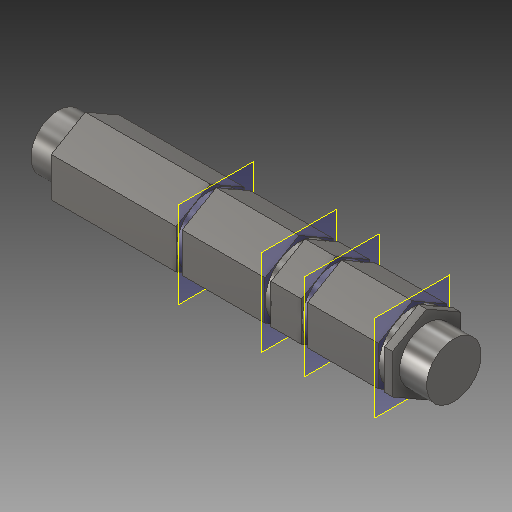
# Autodesk Inventor part: Shaft Jr
Saved by Autodesk Inventor 2019.4 (Build 234330000, 330)
## iProperties
Created: 2019-12-11
Part Number: Shaft Jr
Material: Steel, Mild
Document SubType Name: Modeling
Designer: admin
Density: 7.85 g/cm^3
Appearance: Semi-Polished
Mass: 72.1586 g
Surface Area: 33.9276 cm^2
Volume: 9.19217 cm^3
Author: admin
Autodesk Inventor part; units mm, degrees
ref_plane "YZ Plane" through (0, 0, 0) normal (1, 0, 0) x (0, 1, 0)
ref_plane "XZ Plane" through (0, 0, 0) normal (0, 1, 0) x (-1, 0, 0)
ref_plane "XY Plane" through (0, 0, 0) normal (0, 0, 1) x (1, 0, 0)
sketch "Sketch1" plane through (0, 0, 0) normal (0, 0, 1) x (1, 0, 0)
  line L0 (0, 0) -> (0, 5)
  line L1 (0, 5) -> (5, 5)
  line L2 (5, 5) -> (5, 15)
  line L3 (5, 15) -> (67.6, 15)
  line L4 (67.6, 15) -> (67.6, 5)
  line L5 (67.6, 5) -> (72.6, 5)
  line L6 (72.6, 5) -> (72.6, 0)
  line L7 (72.6, 0) -> (0, 0)
  dimension "d0" = 5
  dimension "d1" = 15
  dimension "d2" = 5
  dimension "d3" = 5
  dimension "d4" = 62.6
  constraints: 16 end point, 6 perpendicular, 2 point on line, 1 vertical
  measures "d0" distance of L5.end L6.end
  measures "d1" distance between parallel lines of L7 L3
  measures "d2" distance of L0.end L1.end
  measures "d3" distance of L4.end L5.end
  measures "d4" distance of L2.end L3.end
revolve "Revolution1" add sketch "Sketch1" angle 360 about axis through (72.6, 0, 0) along (-1, 0, 0)
sketch "Sketch2" plane through (67.6, 0, 0) normal (1, 0, 0) x (0, 0, -1)
  line L0 (0, 7.2169) -> (6.25, 3.6084)
  line L1 (6.25, 3.6084) -> (6.25, -3.6084)
  line L2 (6.25, -3.6084) -> (0, -7.2169)
  line L3 (0, -7.2169) -> (-6.25, -3.6084)
  line L4 (-6.25, -3.6084) -> (-6.25, 3.6084)
  line L5 (-6.25, 3.6084) -> (0, 7.2169)
  circle A0 centre (0, 0) radius 15 projected
  dimension "d6" = 12.5
  constraints: 12 end point, 1 coincident, 13 other
  measures "d6" distance between parallel lines of L1 L4
extrude "Extrusion1" cut sketch "Sketch2" against normal through all
ref_plane "Work Plane1" through (29, -3.6084, -6.25) normal (-1, 0, 0) x (0, 0, 1)
sketch "Sketch3" plane through (29, -3.6084, -6.25) normal (-1, 0, 0) x (0, 0, 1)
  circle A0 centre (6.25, 3.6084) radius 6.2
  line L0 (12.5, 7.2169) -> (6.25, 10.8253) projected
  circle A1 centre (6.25, 3.6084) radius 7.2169
  dimension "d10" = 12.4
  constraints: 2 coincident, 1 centre point, 1 vertical alignment, 2 other
  measures "d10" diameter of A0
extrude "Extrusion2" cut sketch "Sketch3" along normal blind 1.1
ref_plane "Work Plane2" through (44.2, -3.6084, -6.25) normal (-1, 0, 0) x (0, 0, 1)
sketch "Sketch4" plane through (44.2, -3.6084, -6.25) normal (-1, 0, 0) x (0, 0, 1)
  circle A0 centre (6.25, 3.6084) radius 6.2
  line L0 (12.5, 0) -> (12.5, 7.2169) projected
  circle A1 centre (6.25, 3.6084) radius 7.2169
  dimension "d14" = 12.4
  constraints: 2 coincident, 1 centre point, 3 other
  measures "d14" diameter of A0
extrude "Extrusion3" cut sketch "Sketch4" against normal blind 1.1
ref_plane "Work Plane3" through (52, -3.6084, -6.25) normal (-1, 0, 0) x (0, 0, 1)
sketch "Sketch5" plane through (52, -3.6084, -6.25) normal (-1, 0, 0) x (0, 0, 1)
  circle A0 centre (6.25, 3.6084) radius 6.2
  line L0 (12.5, 0) -> (12.5, 7.2169) projected
  circle A1 centre (6.25, 3.6084) radius 7.2169
  dimension "d18" = 12.4
  constraints: 2 coincident, 1 centre point, 3 other
  measures "d18" diameter of A0
extrude "Extrusion4" cut sketch "Sketch5" along normal blind 1.1
ref_plane "Work Plane4" through (65, -3.6084, -6.25) normal (-1, 0, 0) x (0, 0, 1)
sketch "Sketch6" plane through (65, -3.6084, -6.25) normal (-1, 0, 0) x (0, 0, 1)
  circle A0 centre (6.25, 3.6084) radius 6.2
  line L0 (6.25, -3.6084) -> (12.5, 0) projected
  circle A1 centre (6.25, 3.6084) radius 7.2169
  dimension "d22" = 12.4
  constraints: 2 coincident, 1 centre point, 3 other
  measures "d22" diameter of A0
extrude "Extrusion5" cut sketch "Sketch6" against normal blind 1.1
body "Solid1"
